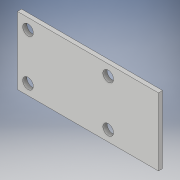
# Autodesk Inventor part: LeftSupportBracket
Saved by Autodesk Inventor 2019.3 (Build 233278000, 278)
## iProperties
Created: 2019-01-26
Part Number: LeftSupportBracket
Material: Generic
Document SubType Name: Modeling
Designer: mark
Density: 1 g/cm^3
Appearance: Default
Author: mark
Autodesk Inventor part; units mm, degrees
ref_plane "YZ Plane" through (0, 0, 0) normal (1, 0, 0) x (0, 1, 0)
ref_plane "XZ Plane" through (0, 0, 0) normal (0, 1, 0) x (-1, 0, 0)
ref_plane "XY Plane" through (0, 0, 0) normal (0, 0, 1) x (1, 0, 0)
sketch "Sketch1" plane through (0, 0, 0) normal (0, 0, 1) x (1, 0, 0)
  line L0 (0, 0) -> (105.92, 0)
  line L1 (105.92, 0) -> (105.92, 50.75)
  line L2 (105.92, 50.75) -> (0, 50.75)
  line L3 (0, 50.75) -> (0, 0)
  circle A0 centre (8, 42.75) radius 4
  circle A1 centre (68.2, 42.75) radius 4
  circle A2 centre (8, 8) radius 4
  circle A3 centre (68.2, 8) radius 4
  dimension "d0" = 105.92
  dimension "d1" = 50.75
  dimension "d2" = 8
  dimension "d3" = 8
  dimension "d4" = 8
  dimension "d5" = 8
  dimension "d6" = 8
  dimension "d7" = 8
  dimension "d8" = 8
  dimension "d9" = 8
  dimension "d10" = 60.2
  dimension "d11" = 60.2
  dimension "d12" = 8
  dimension "d13" = 8
  constraints: 8 end point, 4 centre point, 3 perpendicular, 1 horizontal
  measures "d0" distance of L2.end L1.end
  measures "d1" distance of L1.end L0.end
  measures "d2" diameter of A0
  measures "d3" diameter of A2
  measures "d4" diameter of A1
  measures "d5" diameter of A3
  measures "d6" distance from line of L3 A0.centre
  measures "d7" distance from line of A0.centre L2
  measures "d8" distance from line of L3 A2.centre
  measures "d9" distance from line of A2.centre L0
  measures "d10" distance of A1.centre A0.centre
  measures "d11" distance of A2.centre A3.centre
  measures "d12" distance from line of L2 A1.centre
  measures "d13" distance from line of L0 A3.centre
extrude "Extrusion1" add sketch "Sketch1" along normal blind 3.1
body "Solid1"
